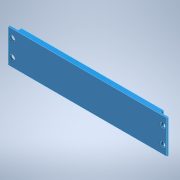
# Autodesk Inventor part: Крышка на ESC
Saved by Autodesk Inventor 2022 (Build 260153000, 153)
## iProperties
Created: 2021-12-26
Part Number: Крышка на ESC
Material: Пластик ПЭТ
Document SubType Name: Modeling
Designer: Grigori
Density: 1.541 g/cm^3
Appearance: Поликарбонат — прозрачный
Author: Grigori
Autodesk Inventor part; units mm, degrees
ref_plane "YZ Plane" through (0, 0, 0) normal (1, 0, 0) x (0, 1, 0)
ref_plane "XZ Plane" through (0, 0, 0) normal (0, 1, 0) x (-1, 0, 0)
ref_plane "XY Plane" through (0, 0, 0) normal (0, 0, 1) x (1, 0, 0)
sketch "Эскиз1" plane through (0, 0, 0) normal (0, 0, 1) x (1, 0, 0)
  point P0 (0, 0)
sketch "Эскиз2" plane through (0, 0, 0) normal (0, 0, 1) x (1, 0, 0)
  line L0 (0, 0) -> (85, 0)
  line L1 (85, 0) -> (85, 20)
  line L2 (85, 20) -> (0, 20)
  line L3 (0, 20) -> (0, 0)
  dimension "d0" = 85
  dimension "d1" = 20
  constraints: 8 end point, 2 parallel, 1 horizontal, 1 perpendicular
  measures "d0" distance of L2.end L1.end
  measures "d1" distance of L1.end L0.end
extrude "Выдавливание1" add sketch "Эскиз2" along normal blind 3
sketch "Эскиз3" plane through (0, 0, 3) normal (0, 0, 1) x (1, 0, 0)
  line L0 (0, 20) -> (0, 0) projected
  line L1 (85, 0) -> (85, 20) projected
  line L2 (0, 20) -> (-5, 20)
  line L3 (-5, 20) -> (-5, 0)
  line L4 (-5, 0) -> (0, 0)
  line L5 (0, 0) -> (0, 20)
  circle A0 centre (-2.5, 15) radius 1.5
  circle A1 centre (-2.5, 5) radius 1.5
  line L6 (85, 20) -> (85, 0)
  line L7 (85, 20) -> (90, 20)
  line L8 (90, 20) -> (90, 0)
  line L9 (90, 0) -> (85, 0)
  line L10 (85, 0) -> (85, 20)
  circle A2 centre (87.5, 15) radius 1.5
  circle A3 centre (87.5, 5) radius 1.5
  dimension "d4" = 5
  dimension "d7" = 3
  dimension "d8" = 3
  constraints: 18 end point, 4 centre point, 2 parallel, 1 horizontal, 1 perpendicular
  measures "d4" distance of L4.end L3.end
  measures "d7" diameter of A0
  measures "d8" diameter of A1
extrude "Выдавливание2" add sketch "Эскиз3" against normal blind 1
